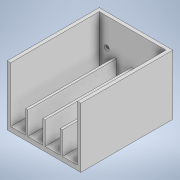
# Autodesk Inventor part: shelfForElectronics
Saved by Autodesk Inventor 2021.2 (Build 252289000, 289)
## iProperties
Created: 2020-12-15
Part Number: shelfForElectronics
Material: Generic
Document SubType Name: Modeling
Designer: robst
Density: 1 g/cm^3
Appearance: Default
Author: robst
Autodesk Inventor part; units mm, degrees
ref_plane "YZ Plane" through (0, 0, 0) normal (1, 0, 0) x (0, 1, 0)
ref_plane "XZ Plane" through (0, 0, 0) normal (0, 1, 0) x (-1, 0, 0)
ref_plane "XY Plane" through (0, 0, 0) normal (0, 0, 1) x (1, 0, 0)
sketch "Sketch2" plane through (0, 0, 0) normal (0, 1, 0) x (-1, 0, 0)
  line L0 (50.8, 63.5) -> (-50.8, 63.5)
  line L1 (-50.8, 63.5) -> (-50.8, -63.5)
  line L2 (-50.8, -63.5) -> (50.8, -63.5)
  line L3 (50.8, -63.5) -> (50.8, 63.5)
  line L4 (50.8, 63.5) -> (-50.8, -63.5) construction
  line L5 (-50.8, 63.5) -> (50.8, -63.5) construction
  point P0 (0, 0)
  dimension "d0" = 127
  dimension "d1" = 101.6
  constraints: 12 end point, 2 midpoint, 2 parallel, 1 horizontal, 1 perpendicular
  measures "d0" distance of L2.end L0.start
  measures "d1" distance of L1.end L2.end
extrude "Extrusion1" add sketch "Sketch2" against normal blind 6.35
sketch "Sketch4" plane through (0, 0, 0) normal (0, 1, 0) x (1, 0, 0)
  line L0 (-50.8, -63.5) -> (-50.8, 63.5) projected
  line L1 (50.8, 63.5) -> (50.8, -63.5) projected
  line L2 (-50.8, 63.5) -> (50.8, 63.5)
  line L3 (50.8, 63.5) -> (50.8, 58.7375)
  line L4 (50.8, 58.7375) -> (-50.8, 58.7375)
  line L5 (-50.8, 58.7375) -> (-50.8, 63.5)
  point P0 (0, 0)
  dimension "d4" = 4.7625
  constraints: 8 end point, 2 parallel, 1 horizontal, 1 perpendicular, 1 point on line
  measures "d4" distance between parallel lines of L4 L2
extrude "Extrusion2" add sketch "Sketch4" along normal blind 76.2
sketch "Sketch5" plane through (0, 0, 0) normal (0, 1, 0) x (1, 0, 0)
  line L0 (50.8, -63.5) -> (-50.8, -63.5) projected
  line L1 (-50.8, 58.7375) -> (50.8, 58.7375) projected
  line L2 (-50.8, -63.5) -> (-46.0375, -63.5)
  line L3 (-46.0375, -63.5) -> (-46.0375, 58.7375)
  line L4 (-46.0375, 58.7375) -> (-50.8, 58.7375)
  line L5 (-50.8, 58.7375) -> (-50.8, -63.5)
  line L6 (50.8, 63.5) -> (50.8, -63.5) projected
  line L7 (50.8, -63.5) -> (46.0375, -63.5)
  line L8 (46.0375, -63.5) -> (46.0375, 58.7375)
  line L9 (46.0375, 58.7375) -> (50.8, 58.7375)
  line L10 (50.8, 58.7375) -> (50.8, -63.5)
  point P0 (0, 0)
  point P1 (46.0375, 58.7375)
  point P2 (46.0375, -63.5)
  dimension "d7" = 4.7625
  dimension "d8" = 4.7625
  constraints: 16 end point, 4 parallel, 2 horizontal, 2 perpendicular, 2 point on line
  measures "d7" distance between parallel lines of L3 L5
  measures "d8" distance between parallel lines of L6 L8
extrude "Extrusion3" add sketch "Sketch5" along normal blind 76.2 contours L0 L8 L1 L6 | L0 L5 L1 L3
sketch "Sketch6" plane through (0, 0, 0) normal (0, 1, 0) x (1, 0, 0)
  line L0 (-46.0375, -63.5) -> (46.0375, -63.5) projected
  line L1 (-46.0375, 58.7375) -> (46.0375, 58.7375) projected
  line L2 (-25.4, -63.5) -> (-22.225, -63.5)
  line L3 (-22.225, -63.5) -> (-22.225, 58.7375)
  line L4 (-22.225, 58.7375) -> (-25.4, 58.7375)
  line L5 (-25.4, 58.7375) -> (-25.4, -63.5)
  line L6 (-1.5875, -63.5) -> (1.5875, -63.5)
  line L7 (1.5875, -63.5) -> (1.5875, 58.7375)
  line L8 (1.5875, 58.7375) -> (-1.5875, 58.7375)
  line L9 (-1.5875, 58.7375) -> (-1.5875, -63.5)
  line L10 (22.225, -63.5) -> (25.4, -63.5)
  line L11 (25.4, -63.5) -> (25.4, 58.7375)
  line L12 (25.4, 58.7375) -> (22.225, 58.7375)
  line L13 (22.225, 58.7375) -> (22.225, -63.5)
  line L14 (-46.0375, -63.5) -> (-46.0375, 58.7375) projected
  line L15 (46.0375, 58.7375) -> (46.0375, -63.5) projected
  point P0 (0, 0)
  point P1 (22.225, -63.5)
  point P2 (25.4, -63.5)
  point P3 (25.4, 58.7375)
  point P4 (-1.5875, 58.7375)
  point P5 (-1.5875, -63.5)
  point P6 (-22.225, -63.5)
  dimension "d11" = 3.175
  dimension "d12" = 3.175
  dimension "d13" = 3.175
  dimension "d14" = 20.6375
  dimension "d15" = 20.6375
  dimension "d16" = 20.6375
  dimension "d17" = 20.6375
  constraints: 24 end point, 6 parallel, 6 point on line, 3 horizontal, 3 perpendicular
  measures "d11" distance between parallel lines of L3 L5
  measures "d12" distance between parallel lines of L7 L9
  measures "d13" distance between parallel lines of L11 L13
  measures "d14" distance between parallel lines of L9 L3
  measures "d15" distance between parallel lines of L13 L7
  measures "d16" distance between parallel lines of L5 L14
  measures "d17" distance between parallel lines of L11 L15
extrude "Extrusion4" add sketch "Sketch6" along normal blind 31.75 contours L5 L1 L3 L0 | L9 L1 L7 L0 | L13 L1 L11 L0
sketch "Sketch7" plane through (-46.0375, 0, -58.7375) normal (0, 0, 1) x (1, 0, 0)
  line L0 (0, 76.2) -> (0, 0) construction
  line L1 (0, 38.1) -> (92.075, 38.1) construction
  line L2 (92.075, 0) -> (92.075, 76.2) construction
  line L3 (46.0375, 38.1) -> (46.0375, 76.2) construction
  line L4 (96.8375, 76.2) -> (-4.7625, 76.2) construction
  point P0 (46.0375, 0)
  point P1 (10.3187, 38.1)
  point P2 (81.7562, 38.1)
  dimension "d18" = 10.3187
  constraints: 4 end point, 4 midpoint, 1 point on line, 1 symmetric about line
  measures "d18" distance from line of point (10.319, 38.1) L0
hole "Hole1" at (-35.7188, 38.1, -58.7375) at (35.7187, 38.1, -58.7375) direction (0, 0, -1) diameter 3.81 end through all countersink diameter 7.0866 countersink angle 82 clearance for "Flat Head Machine Screw (82)" size "#6" standard "Ansi Unified Screw Threads"
equation "\"d0\" = depth"
equation "\"d1\" = width"
equation "\"d2\" = baseThickness"
equation "\"d4\" = backThickness"
equation "\"d5\" = backHeight"
equation "\"d7\" = edgeThickness"
equation "\"d8\" = edgeThickness"
equation "\"d9\" = edgeHeight"
equation "\"d11\" = dividerThickness"
equation "\"d12\" = dividerThickness"
equation "\"d13\" = dividerThickness"
equation "\"d14\" = dividerGap"
equation "\"d15\" = dividerGap"
equation "\"d16\" = dividerGap"
equation "\"d18\" = 0.5 * dividerGap"
equation "\"baseThickness\" = 6.35"
equation "\"width\" = 101.6"
equation "\"depth\" = 127"
equation "\"backHeight\" = 76.2"
equation "\"backThickness\" = 4.7625"
equation "\"edgeThickness\" = 4.7625"
equation "\"edgeHeight\" = 76.2"
equation "\"dividerThickness\" = 3.175"
equation "\"dividerHeight\" = 31.75"
equation "\"dividerGap\" = 20.6375"
body "Solid1"
